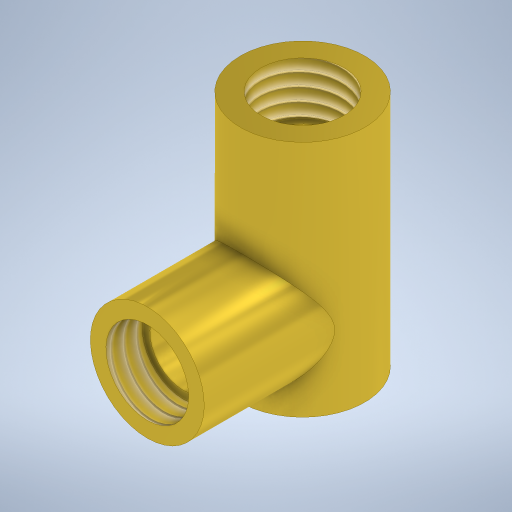
# Autodesk Inventor part: HUDSON-1-88
Saved by Autodesk Inventor 2024.2 (Build 282272000, 272)
## iProperties
Created: 2024-09-29
Part Number: HUDSON-1-88
Material: Generic
Document SubType Name: Modeling
Designer: melim
Density: 1 g/cm^3
Appearance: Metal 2400F Hot
Author: melim
Autodesk Inventor part; units mm, degrees
ref_plane "YZ Plane" through (0, 0, 0) normal (1, 0, 0) x (0, 1, 0)
ref_plane "XZ Plane" through (0, 0, 0) normal (0, 1, 0) x (-1, 0, 0)
ref_plane "XY Plane" through (0, 0, 0) normal (0, 0, 1) x (1, 0, 0)
sketch "Sketch4" plane through (0, 0, 0) normal (0, 0, 1) x (1, 0, 0)
  line L0 (0, -13.961) -> (0, 29.8829)
  line L1 (0, 0) -> (-6, 0)
  line L2 (-6, 0) -> (-6, 23)
  line L3 (-6, 23) -> (-4, 23)
  line L4 (-4, 23) -> (-4, 18)
  line L5 (-4, 18) -> (-3.25, 18)
  line L6 (-3.25, 18) -> (-3.25, 12)
  line L7 (-3.25, 12) -> (-2.25, 12)
  line L8 (-2.25, 12) -> (-2.25, 0)
  point P0 (-4, 20.5)
  dimension "d18" = 12
  dimension "d19" = 23
  dimension "d21" = 8
  dimension "d22" = 5
  dimension "d23" = 6.5
  dimension "d24" = 11
  dimension "d26" = 4.5
  constraints: 18 end point, 4 perpendicular, 3 vertical, 2 point on line, 1 horizontal, 1 midpoint
  measures "d18" diameter of L1.end L0
  measures "d19" distance of L1.end L2.end
  measures "d21" diameter of point (-4, 20.5) L0
  measures "d22" distance of L3.end L4.end
  measures "d23" diameter of L6 L0
  measures "d24" distance between parallel lines of L3 L7
  measures "d26" diameter of L8 L0
revolve "Revolution1" add sketch "Sketch4" angle 360 about axis through (0, -13.961, 0) along (0, 1, 0)
thread "Thread1" size "M8x1.25" class "6H" standard "ANSI Metric M Profile" full length
sketch "Sketch5" plane through (0, 0, 0) normal (1, 0, 0) x (0, 1, 0)
  line L0 (7, 2) -> (7, 20.6305)
  line L1 (0, -6) -> (0, 6) projected
  line L2 (0, -6) -> (0, 6) projected
  line L3 (23, -6) -> (23, 6) projected
  line L4 (7, 15) -> (1.5, 15)
  line L5 (3, 15) -> (3, 11.5)
  line L6 (3, 11.5) -> (7, 11.5)
  line L7 (3.75, 11.5) -> (3.75, 8)
  line L8 (3.75, 8) -> (7, 8)
  line L9 (5.25, 8) -> (5.25, 2)
  line L10 (12, 2.25) -> (0, 2.25) projected
  line L11 (1.5, 2) -> (7, 2)
  line L12 (1.5, 15) -> (1.5, 6)
  line L13 (1.5, 6) -> (1.5, 2)
  line L14 (0, 6) -> (23, 6) projected
  line L15 (7, 6) -> (0, 6)
  point P0 (0, 0)
  dimension "d30" = 7
  dimension "d34" = 11
  dimension "d35" = 8
  dimension "d36" = 3.5
  dimension "d37" = 7
  dimension "d38" = 6.5
  dimension "d39" = 3.5
  dimension "d43" = 9
  dimension "d44" = 4
  dimension "d45" = 4
  constraints: 22 end point, 10 point on line, 4 vertical, 3 perpendicular, 1 collinear, 1 horizontal
  measures "d30" distance from line of point (0, 0) L0
  measures "d34" diameter of L4.end L0
  measures "d35" diameter of L5 L0
  measures "d36" distance of L5.start L5.end
  measures "d37" distance between parallel lines of L4 L8
  measures "d38" diameter of L7 L0
  measures "d39" diameter of L9 L0
  measures "d43" distance of L4.end L12.end
  measures "d44" distance from line of L15 L9.end
  measures "d45" distance from line of L11.start L15
revolve "Revolution4" add sketch "Sketch5" angle 360 about axis through (0, 7, 2) along (0, 0, 1) contours L14 L12 L4 L5 L6 L7 L8 L9 | L9 L10 L13 L14 | L9 L11 L13 L10
sketch "Sketch6" plane through (0, 23, 0) normal (0, 1, 0) x (1, 0, 0)
  point P0 (0, 0)
hole "Hole3" at (0, 23, 0) direction (0, -1, 0) diameter 4.5 end through all counterbore diameter 6.5 counterbore depth 11
sketch "Sketch7" plane through (0, 7, 15) normal (0, 0, 1) x (1, 0, 0)
  circle A0 centre (0, 0) radius 5.5 projected
  circle A1 centre (0, 0) radius 4 projected
  circle A2 centre (0, 0) radius 3.25 projected
  circle A3 centre (0, 0) radius 1.75 projected
  point P0 (0, -7)
  constraints: 1 other
hole "Hole4" at (0, 7, 15) direction (0, 0, -1) diameter 3.5 end up to surface counterbore diameter 6.5 counterbore depth 7
thread "Thread2" size "M8x1.25" class "6H" standard "ANSI Metric M Profile" full length
body "Solid2"
